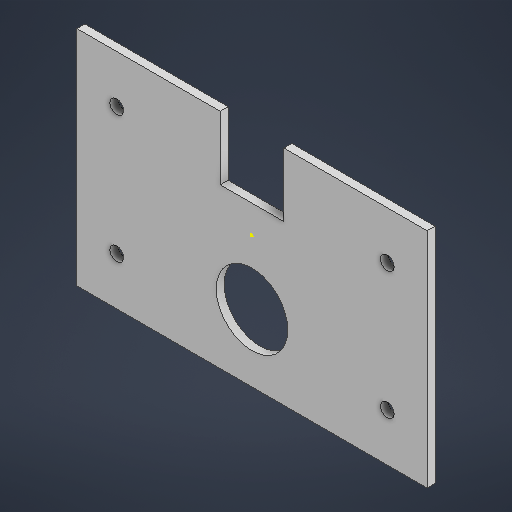
# Autodesk Inventor part: DIFF_PLATE_ROD
Saved by Autodesk Inventor 2026.1 (Build 301233020, 233B)
## iProperties
Created: 2024-01-10
Part Number: DIFF_PLATE_ROD
Material: Generic
Document SubType Name: Modeling
Designer: bugme
Density: 1 g/cm^3
Appearance: Default
Author: bugme
Autodesk Inventor part; units mm, degrees
ref_plane "YZ Plane" through (0, 0, 0) normal (1, 0, 0) x (0, 1, 0)
ref_plane "XZ Plane" through (0, 0, 0) normal (0, 1, 0) x (-1, 0, 0)
ref_plane "XY Plane" through (0, 0, 0) normal (0, 0, 1) x (1, 0, 0)
sketch "Sketch1" plane through (0, 0, 0) normal (0, 0, 1) x (1, 0, 0)
  line L0 (0, -70.231) -> (0, 54.229) projected
  line L1 (69.85, 36.449) -> (69.85, -52.451)
  line L2 (69.85, -52.451) -> (-69.85, -52.451)
  line L3 (-69.85, -52.451) -> (-69.85, 36.449)
  line L4 (-97.79, 0) -> (97.79, 0) projected
  line L5 (-12.7, 36.449) -> (-12.7, 11.049)
  line L6 (-12.7, 11.049) -> (12.7, 11.049)
  line L7 (12.7, 11.049) -> (12.7, 36.449)
  line L8 (-69.85, 36.449) -> (-12.7, 36.449)
  line L9 (12.7, 36.449) -> (69.85, 36.449)
  line L10 (0, -52.451) -> (0, -25.654)
  circle A0 centre (0, -25.654) radius 14.2875
  point P0 (0, 0)
  dimension "d0" = 139.7
  dimension "d1" = 88.9
  dimension "d2" = 25.4
  dimension "d3" = 25.4
  dimension "d5" = 28.575
  dimension "d21" = 62.103
  constraints: 18 end point, 4 perpendicular, 2 horizontal, 2 vertical, 1 centre point, 1 coincident, 1 midpoint, 1 point on line, 1 symmetric about line, 1 other
  measures "d0" distance of L3.end L1.start
  measures "d1" distance of L1.start L1.end
  measures "d2" distance of L5.start L5.end
  measures "d3" distance of L5.end L6.end
  measures "d5" diameter of A0
  measures "d21" distance from line of A0.centre L8
extrude "Extrusion1" add sketch "Sketch1" along normal blind 3.175 contours L2 L3 L4 L0 A0 | L0 A0 L4 L1 L2 | L4 L0 L6 L7 L9 L1 | L3 L8 L5 L6 L0 L4
sketch "Sketch2" plane through (0, 0, 3.175) normal (0, 0, 1) x (1, 0, 0)
  line L0 (69.85, -52.451) -> (69.85, 36.449) projected
  line L1 (-69.85, -52.451) -> (69.85, -52.451) projected
  line L2 (69.85, 36.449) -> (12.7, 36.449) projected
  point P0 (0, 0)
  point P1 (53.975, 17.399)
  point P2 (53.975, -33.401)
  point P3 (53.975, 38.643)
  dimension "d16" = 15.875
  dimension "d18" = 19.05
  dimension "d20" = 19.05
  constraints: 2 vertical alignment
  measures "d16" distance from line of L0 point (53.975, 17.399)
  measures "d18" distance from line of L1 point (53.975, -33.401)
  measures "d20" distance from line of point (53.975, 17.399) L2
hole "Hole1" at (53.975, 17.399, 3.175) at (53.975, -33.401, 3.175) direction (0, 0, -1) diameter 5.5118 end through all clearance for "Flat Head Machine Screw" size "M5" standard "Ansi Metric M Profile"
mirror "Mirror1" about plane through (0, 0, 0) normal (1, 0, 0) of "Hole1"
sketch "Sketch3" plane through (0, 0, 3.175) normal (0, 0, 1) x (1, 0, 0)
  point P0 (0, 0)
equation "\"d20\" = d18"
body "Solid1"
